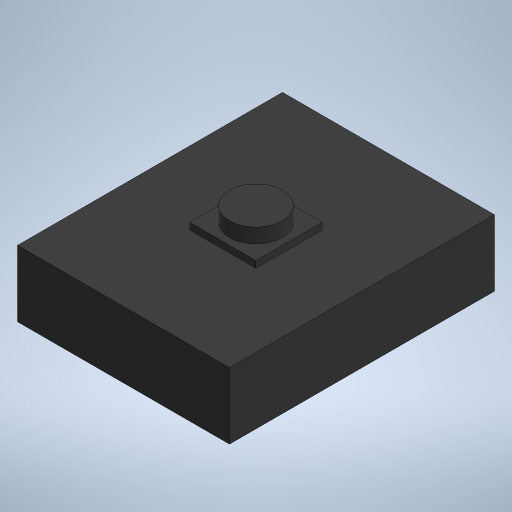
# Autodesk Inventor part: Force_sensor
Saved by Autodesk Inventor 2024 (Build 280153000, 153)
## iProperties
Created: 2025-02-15
Part Number: Force_sensor
Material: Generic
Document SubType Name: Modeling
Designer: XxPan
Density: 1 g/cm^3
Appearance: Default
Author: XxPan
Autodesk Inventor part; units mm, degrees
ref_plane "YZ Plane" through (0, 0, 0) normal (1, 0, 0) x (0, 1, 0)
ref_plane "XZ Plane" through (0, 0, 0) normal (0, 1, 0) x (-1, 0, 0)
ref_plane "XY Plane" through (0, 0, 0) normal (0, 0, 1) x (1, 0, 0)
sketch "Sketch1" plane through (0, 0, 0) normal (0, 1, 0) x (-1, 0, 0)
  line L0 (0.8, 1) -> (-0.8, 1)
  line L1 (-0.8, 1) -> (-0.8, -1)
  line L2 (-0.8, -1) -> (0.8, -1)
  line L3 (0.8, -1) -> (0.8, 1)
  line L4 (1.12, 0) -> (-1.12, 0) construction
  line L5 (0, -1.4) -> (0, 1.4) construction
  point P0 (0, 0)
  point P1 (0.8, 0)
  point P2 (0, 1)
  dimension "d0" = 1.6
  dimension "d1" = 2
  constraints: 8 end point, 2 midpoint, 2 parallel, 2 point on line, 1 horizontal, 1 perpendicular
  measures "d0" distance of L2.end L1.end
  measures "d1" distance of L1.end L0.end
extrude "Extrusion1" add sketch "Sketch1" along normal blind 0.5
sketch "Sketch2" plane through (0, 0.5, 0) normal (0, 1, 0) x (1, 0, 0)
  circle A0 centre (0, 0) radius 0.2
  line L0 (-0.25, -0.25) -> (0.25, -0.25)
  line L1 (0.25, -0.25) -> (0.25, 0.25)
  line L2 (0.25, 0.25) -> (-0.25, 0.25)
  line L3 (-0.25, 0.25) -> (-0.25, -0.25)
  line L4 (-1.12, 0) -> (1.12, 0) construction
  line L5 (0, 1.4) -> (0, -1.4) construction
  point P0 (-0.25, 0)
  point P1 (0, -0.25)
  dimension "d4" = 0.4
  dimension "d5" = 0.5
  dimension "d6" = 0.5
  constraints: 8 end point, 2 midpoint, 2 parallel, 2 point on line, 1 centre point, 1 coincident, 1 horizontal, 1 perpendicular
  measures "d4" diameter of A0
  measures "d5" distance of L2.end L1.end
  measures "d6" distance of L1.end L0.end
extrude "Extrusion2" add sketch "Sketch2" along normal blind 0.05
extrude "Extrusion3" add sketch "Sketch2" along normal blind 0.16 contours A0
body "Solid1"
